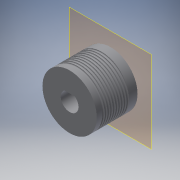
# Autodesk Inventor part: big one
Saved by Autodesk Inventor 2019 (Build 230136000, 136)
## iProperties
Created: 2021-03-26
Part Number: big one
Material: Generic
Document SubType Name: Modeling
Designer: Ian
Density: 1 g/cm^3
Appearance: Default
Author: Ian
Autodesk Inventor part; units mm, degrees
ref_plane "YZ Plane" through (0, 0, 0) normal (1, 0, 0) x (0, 1, 0)
ref_plane "XZ Plane" through (0, 0, 0) normal (0, 1, 0) x (-1, 0, 0)
ref_plane "XY Plane" through (0, 0, 0) normal (0, 0, 1) x (1, 0, 0)
ref_plane "Work Plane1" through (0, 0, 0.1) normal (0, 0, 1) x (1, 0, 0)
sketch "Sketch1" plane through (0, 0, 0.1) normal (0, 0, 1) x (1, 0, 0)
  circle A0 centre (0, 0) radius 8
  line L0 (1.5, 2) -> (-1.5, 2) projected
  arc A1 (-1.5, 2) -> (1.5, 2) centre (0, 0) ccw projected
  line L1 (-1.5411, 2.125) -> (1.5411, 2.125)
  arc A2 (-1.5411, 2.125) -> (1.5411, 2.125) centre (0, 0) ccw
  circle A3 centre (0, 0) radius 2.625 construction
  line L2 (-0.7133, 3.975) -> (1.2496, 3.975) construction
  line L3 (1.2496, 3.975) -> (1.2496, 3.375) construction
  line L4 (1.2496, 3.375) -> (-0.5971, 3.375) construction
  dimension "d1" = 0.125
  dimension "d18" = 0.6
  dimension "d35" = 16
  constraints: 8 end point, 3 centre point, 2 concentric, 2 perpendicular, 2 point on circle, 1 coincident, 1 horizontal, 1 other
  measures "d1" distance between parallel lines of L0 L1
  measures "d18" distance between parallel lines of L4 L2
  measures "d35" diameter of A0
extrude "Extrusion1" add sketch "Sketch1" along normal blind 12 contours A0
sketch "Sketch5" plane through (0, 0, 0) normal (1, 0, 0) x (0, 1, 0)
  line L0 (21, 1) -> (8.4705, 1) construction
  line L1 (8.4705, 1) -> (-14.7037, 1) construction
  line L2 (8, 0.1) -> (8, 12.1) projected
  line L3 (7.9, 10.45) -> (8, 10.45)
  line L4 (8, 10.45) -> (8, 9.85)
  line L5 (8, 0.1) -> (8, 12.1) projected
  line L6 (8, 9.85) -> (7.9, 9.85)
  line L7 (8, 12.1) -> (-8, 12.1) projected
  arc A0 (7.9, 10.45) -> (7.9, 9.85) centre (7.9, 10.15) ccw
  arc A1 (7.9, 9.65) -> (7.9, 9.05) centre (7.9, 9.35) ccw
  line L8 (7.9, 9.65) -> (8, 9.65)
  line L9 (8, 9.65) -> (8, 9.05)
  line L10 (8, 9.05) -> (7.9, 9.05)
  arc A2 (7.9, 8.85) -> (7.9, 8.25) centre (7.9, 8.55) ccw
  line L11 (7.9, 8.85) -> (8, 8.85)
  line L12 (8, 8.85) -> (8, 8.25)
  line L13 (8, 8.25) -> (7.9, 8.25)
  arc A3 (7.9, 8.05) -> (7.9, 7.45) centre (7.9, 7.75) ccw
  line L14 (7.9, 8.05) -> (8, 8.05)
  line L15 (8, 8.05) -> (8, 7.45)
  line L16 (8, 7.45) -> (7.9, 7.45)
  arc A4 (7.9, 7.25) -> (7.9, 6.65) centre (7.9, 6.95) ccw
  line L17 (7.9, 7.25) -> (8, 7.25)
  line L18 (8, 7.25) -> (8, 6.65)
  line L19 (8, 6.65) -> (7.9, 6.65)
  arc A5 (7.9, 6.45) -> (7.9, 5.85) centre (7.9, 6.15) ccw
  line L20 (7.9, 6.45) -> (8, 6.45)
  line L21 (8, 6.45) -> (8, 5.85)
  line L22 (8, 5.85) -> (7.9, 5.85)
  arc A6 (7.9, 5.65) -> (7.9, 5.05) centre (7.9, 5.35) ccw
  line L23 (7.9, 5.65) -> (8, 5.65)
  line L24 (8, 5.65) -> (8, 5.05)
  line L25 (8, 5.05) -> (7.9, 5.05)
  arc A7 (7.9, 4.85) -> (7.9, 4.25) centre (7.9, 4.55) ccw
  line L26 (7.9, 4.85) -> (8, 4.85)
  line L27 (8, 4.85) -> (8, 4.25)
  line L28 (8, 4.25) -> (7.9, 4.25)
  arc A8 (7.9, 4.05) -> (7.9, 3.45) centre (7.9, 3.75) ccw
  line L29 (7.9, 4.05) -> (8, 4.05)
  line L30 (8, 4.05) -> (8, 3.45)
  line L31 (8, 3.45) -> (7.9, 3.45)
  arc A9 (7.9, 3.25) -> (7.9, 2.65) centre (7.9, 2.95) ccw
  line L32 (7.9, 3.25) -> (8, 3.25)
  line L33 (8, 3.25) -> (8, 2.65)
  line L34 (8, 2.65) -> (7.9, 2.65)
  line L35 (0, -2.42) -> (0, 14.52) projected
  point P0 (0, 0)
  dimension "d75" = 0.1
  dimension "d76" = 1.95
  dimension "d77" = 0.3
  dimension "d80" = 0.8
  dimension "d86" = 1.95
  constraints: 62 end point, 20 point on circle, 10 centre point, 3 point on line, 2 perpendicular, 2 tangent, 1 vertical, 81 other
  measures "d75" distance from line of L2 A0.centre
  measures "d76" distance from line of L7 A0.centre
  measures "d77" radius of A0
  measures "d80" distance of A0.centre A1.centre
  measures "d86" distance from line of L1 A9.centre
revolve "Revolution4" cut sketch "Sketch5" angle 360 about axis through (0, 0, -10) along (0, 0, 1)
sketch "Sketch6" plane through (0, 0, 12.1) normal (0, 0, 1) x (1, 0, 0)
  circle A0 centre (0, 0) radius 2.625 projected
  line L0 (-1.5411, 2.125) -> (1.5411, 2.125) projected
  point P0 (0, 0)
  dimension "d53" = 1.125
  dimension "d54" = 0.25
  dimension "d55" = 2
  dimension "d56" = 1
  dimension "d57" = 0.25
  dimension "d58" = 1
  dimension "d62" = 80
  constraints: 22 end point, 7 point on line, 3 equal length, 1 collinear, 1 horizontal, 1 midpoint, 1 parallel, 1 vertical
sketch "Sketch3" plane through (0, 0, 12.1) normal (0, 0, 1) x (1, 0, 0)
  circle A0 centre (0, 0) radius 8 projected
  line L0 (-0.2046, 7.8333) -> (0.3721, 7.8333) construction
  line L1 (0, 7.8333) -> (-0.5956, 6.8073)
  line L2 (0, 7.8333) -> (0.5956, 6.8073)
  line L3 (0, 0) -> (-0.5956, 6.8073)
  line L4 (0, 0) -> (0.5956, 6.8073)
  circle A1 centre (0, 0) radius 6.8333 projected
  dimension "d46" = 10
  dimension "d60" = 1
  constraints: 10 end point, 2 point on circle, 1 equal length, 1 horizontal, 1 point on line, 1 vertical alignment
  measures "d46" angle of L3 L4
  measures "d60" distance edge to line of A1 L0
equation "\"d76\" = d86"
body "Solid1"
